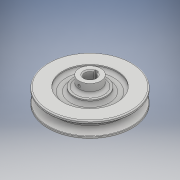
# Autodesk Inventor part: 도면2-4번
Saved by Autodesk Inventor 2018.3 (Build 223284000, 284)
## iProperties
Created: 2019-10-11
Part Number: 도면2-4번
Material: 일반
Document SubType Name: Modeling
Designer: MyTool
Density: 1 g/cm^3
Appearance: 기본값
Author: MyTool
Autodesk Inventor part; units mm, degrees
ref_plane "YZ Plane" through (0, 0, 0) normal (1, 0, 0) x (0, 1, 0)
ref_plane "XZ Plane" through (0, 0, 0) normal (0, 1, 0) x (-1, 0, 0)
ref_plane "XY Plane" through (0, 0, 0) normal (0, 0, 1) x (1, 0, 0)
sketch "스케치1" plane through (0, 0, 0) normal (1, 0, 0) x (0, 1, 0)
  line L0 (38.7, -4.8773) -> (36, -4)
  line L1 (36, -4) -> (29.7, -1.953)
  line L2 (29.7, -1.953) -> (29.7, 0)
  line L3 (29.7, 0) -> (0, 0)
  line L4 (38.7, -4.8773) -> (38.7, -7.5)
  line L5 (38.7, -7.5) -> (0, -7.5)
  line L6 (0, -7.5) -> (0, 0)
  dimension "d1" = 7.5
  dimension "d3" = 72
  dimension "d4" = 18
  dimension "d5" = 4
  dimension "d6" = 2.7
  dimension "d7" = 6.3
  constraints: 14 end point, 3 vertical, 2 perpendicular, 1 collinear
  measures "d1" distance of L5.end L3.end
  measures "d3" diameter of L0.end L6
  measures "d4" angle of L3 L1
  measures "d5" distance from line of L3 L0.end
  measures "d6" horizontal distance of L0.end L0.start
  measures "d7" horizontal distance of L1.end L0.end
revolve "회전1" add sketch "스케치1" angle 360 about axis through (0, 0, -7.5) along (0, 0, 1)
fillet "모깎기1" radius 0.5 1 edges at (0, -38.7, -4.8773)
fillet "모깎기2" radius 1 2 edges at (0, -29.7, -1.953) (0, -38.7, -7.5)
mirror "미러1" about plane through (0, 29.7, 0) normal (0, 0, 1) of "회전1", "모깎기2", "모깎기1"
sketch "스케치2" plane through (0, 0, 7.5) normal (0, 0, 1) x (1, 0, 0)
  circle A0 centre (0, 0) radius 10
  dimension "d11" = 20
  constraints: 1 centre point, 1 coincident
  measures "d11" diameter of A0
extrude "돌출1" add sketch "스케치2" along normal blind 9.5
sketch "스케치3" plane through (0, 0, 17) normal (0, 0, 1) x (1, 0, 0)
  circle A0 centre (0, 0) radius 5
  line L0 (-1.5, 6.4) -> (1.5, 6.4)
  line L1 (1.5, 6.4) -> (1.5, 0)
  line L2 (1.5, 0) -> (-1.5, 0)
  line L3 (-1.5, 0) -> (-1.5, 6.4)
  point P0 (0, 0)
  dimension "d14" = 10
  dimension "d15" = 3
  dimension "d16" = 1.5
  dimension "d17" = 1.4
  constraints: 8 end point, 2 parallel, 1 centre point, 1 coincident, 1 horizontal, 1 perpendicular
  measures "d14" diameter of A0
  measures "d15" distance of L1.end L2.end
  measures "d16" distance from line of point (0, 0) L3
  measures "d17" distance edge to line of A0 L0
extrude "돌출2" cut sketch "스케치3" against normal up to next
chamfer "모따기1" distance 1 angle 45 2 edges at (0, -5, 17) (0, -5, -7.5)
sketch "스케치4" plane through (0, 0, 7.5) normal (0, 0, 1) x (1, 0, 0)
  circle A0 centre (0, 0) radius 15
  circle A1 centre (0, 0) radius 25
  dimension "d23" = 30
  dimension "d24" = 50
  constraints: 2 centre point, 2 coincident
  measures "d23" diameter of A0
  measures "d24" diameter of A1
extrude "돌출3" cut sketch "스케치4" against normal blind 4
mirror "미러2" about plane through (0, 0, 0) normal (0, 0, 1) of "돌출3"
fillet "모깎기3" radius 3 5 edges at (-25, 0, 3.5) (-15, 0, 3.5) (-15, 0, -3.5) (-25, 0, -3.5) (-10, 0, 7.5)
sketch "스케치5" plane through (0, 0, 0) normal (0, 1, 0) x (-1, 0, 0)
  circle A0 centre (0, 13) radius 1.5
  line L0 (6, 17) -> (-6, 17) projected
  point P0 (0, 0)
  point P1 (1.5, 17)
  point P2 (-1.5, 17)
  dimension "d28" = 3
  dimension "d36" = 4
  constraints: 1 centre point
  measures "d28" diameter of A0
  measures "d36" distance from line of A0.centre L0
hole "구멍1" at (0, 0, 13) direction (0, -1, 0) diameter 2.459 end through all thread size "M3x0.5" class "6H" standard "ANSI Metric M Profile"
equation "\"d16\" = 0.5 * d15"
